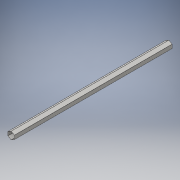
# Autodesk Inventor part: Pencil Outside
Saved by Autodesk Inventor 2016 (Build 200138000, 138)
## iProperties
Created: 2015-08-30
Part Number: Pencil Outside
Material: Generic
Document SubType Name: Modeling
Density: 1 g/cm^3
Appearance: Default
Autodesk Inventor part; units mm, degrees
ref_plane "YZ Plane" through (0, 0, 0) normal (1, 0, 0) x (0, 1, 0)
ref_plane "XZ Plane" through (0, 0, 0) normal (0, 1, 0) x (-1, 0, 0)
ref_plane "XY Plane" through (0, 0, 0) normal (0, 0, 1) x (1, 0, 0)
sketch "Sketch1" plane through (0, 0, 0) normal (0, 1, 0) x (-1, 0, 0)
  line L0 (-2.5, 1.4434) -> (0, 2.8868)
  line L1 (0, 2.8868) -> (2.5, 1.4434)
  line L2 (2.5, 1.4434) -> (2.5, -1.4434)
  line L3 (2.5, -1.4434) -> (0, -2.8868)
  line L4 (0, -2.8868) -> (-2.5, -1.4434)
  line L5 (-2.5, -1.4434) -> (-2.5, 1.4434)
  line L6 (-2.45, 1.4145) -> (0, 2.829)
  line L7 (0, 2.829) -> (2.45, 1.4145)
  line L8 (2.45, 1.4145) -> (2.45, -1.4145)
  line L9 (2.45, -1.4145) -> (0, -2.829)
  line L10 (0, -2.829) -> (-2.45, -1.4145)
  line L11 (-2.45, -1.4145) -> (-2.45, 1.4145)
  point P0 (0, 0)
  point P1 (0, 0)
  point P2 (0, 0)
  dimension "d0" = 5
  dimension "d1" = 4.9
  constraints: 24 end point, 2 coincident, 26 other
  measures "d0" distance between parallel lines of L2 L5
  measures "d1" distance between parallel lines of L8 L11
extrude "Extrusion1" add sketch "Sketch1" along normal blind 120
fillet "Fillet1" radius 0.1 6 edges at (0, 60, 2.8868) (2.5, 60, -1.4434) (0, 60, -2.8868) (-2.5, 60, -1.4434) (-2.5, 60, 1.4434) (2.5, 60, 1.4434)
body "Solid1"
